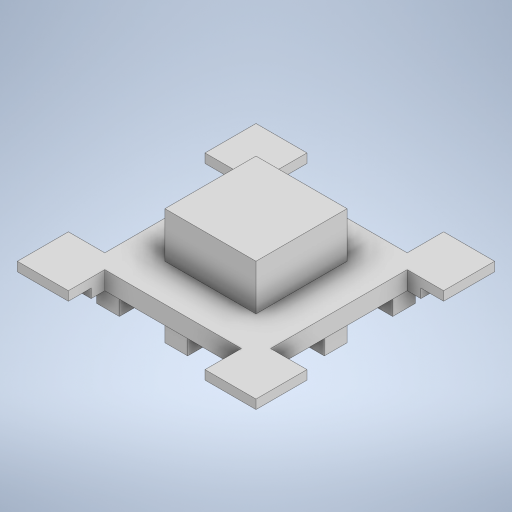
# Autodesk Inventor part: sensor_holder
Saved by Autodesk Inventor 2023.1 (Build 271208000, 208)
## iProperties
Created: 2022-08-08
Part Number: sensor_holder
Material: Generic
Document SubType Name: Modeling
Designer: fraaw
Density: 1 g/cm^3
Appearance: Default
Author: fraaw
## iProperties of the stored document sensor_holder_3DPrint.ipt
Created: 2022-08-08
Part Number: sensor_holder_3DPrint
Material: Generic
Document SubType Name: Modeling
Designer: fraaw
Density: 1 g/cm^3
Appearance: Default
Author: fraaw
Autodesk Inventor part; units mm, degrees
ref_plane "YZ Plane" through (0, 0, 0) normal (1, 0, 0) x (0, 1, 0)
ref_plane "XZ Plane" through (0, 0, 0) normal (0, 1, 0) x (-1, 0, 0)
ref_plane "XY Plane" through (0, 0, 0) normal (0, 0, 1) x (1, 0, 0)
sketch "Sketch1" plane through (0, 0, 0) normal (0, 1, 0) x (-1, 0, 0)
  line L0 (13.1, 13.1) -> (-13.1, 13.1)
  line L1 (-13.1, 13.1) -> (-13.1, -13.1)
  line L2 (-13.1, -13.1) -> (13.1, -13.1)
  line L3 (13.1, -13.1) -> (13.1, 13.1)
  line L4 (13.1, 13.1) -> (-13.1, -13.1) construction
  line L5 (-13.1, 13.1) -> (13.1, -13.1) construction
  point P0 (0, 0)
  dimension "d0" = 26.2
  dimension "d1" = 26.2
  constraints: 12 end point, 2 midpoint, 2 parallel, 1 horizontal, 1 perpendicular
  measures "d0" distance of L1.end L2.end
  measures "d1" distance of L2.end L0.start
extrude "Extrusion1" add sketch "Sketch1" along normal blind 1
sketch "Sketch3" plane through (0, 0, 0) normal (0, -1, 0) x (1, 0, 0)
  line L0 (-10.75, -10.75) -> (10.75, -10.75) construction
  line L1 (10.75, -10.75) -> (10.75, 10.75) construction
  line L2 (10.75, 10.75) -> (-10.75, 10.75) construction
  line L3 (-10.75, 10.75) -> (-10.75, -10.75) construction
  line L4 (-10.75, -10.75) -> (10.75, 10.75) construction
  line L5 (10.75, -10.75) -> (-10.75, 10.75) construction
  line L6 (-10.75, 10.75) -> (-4.25, 10.75) construction
  line L7 (-4.25, 10.75) -> (-4.25, 4.25) construction
  line L8 (-4.25, 4.25) -> (-10.75, 4.25) construction
  line L9 (-10.75, 4.25) -> (-10.75, 10.75) construction
  line L10 (-6.25, 6.25) -> (-8.75, 6.25)
  line L11 (-8.75, 6.25) -> (-8.75, 8.75)
  line L12 (-8.75, 8.75) -> (-6.25, 8.75)
  line L13 (-6.25, 8.75) -> (-6.25, 6.25)
  line L14 (-6.25, 6.25) -> (-8.75, 8.75) construction
  line L15 (-8.75, 6.25) -> (-6.25, 8.75) construction
  line L16 (-1.25, 8.75) -> (1.25, 8.75)
  line L17 (-1.25, 6.25) -> (-1.25, 8.75)
  line L18 (1.25, 6.25) -> (-1.25, 6.25)
  line L19 (1.25, 8.75) -> (1.25, 6.25)
  line L20 (6.25, 8.75) -> (8.75, 8.75)
  line L21 (6.25, 6.25) -> (6.25, 8.75)
  line L22 (8.75, 6.25) -> (6.25, 6.25)
  line L23 (8.75, 8.75) -> (8.75, 6.25)
  line L24 (-8.75, 1.25) -> (-6.25, 1.25)
  line L25 (-8.75, -1.25) -> (-8.75, 1.25)
  line L26 (-6.25, -1.25) -> (-8.75, -1.25)
  line L27 (-6.25, 1.25) -> (-6.25, -1.25)
  line L28 (-1.25, 1.25) -> (1.25, 1.25)
  line L29 (-1.25, -1.25) -> (-1.25, 1.25)
  line L30 (1.25, -1.25) -> (-1.25, -1.25)
  line L31 (1.25, 1.25) -> (1.25, -1.25)
  line L32 (6.25, 1.25) -> (8.75, 1.25)
  line L33 (6.25, -1.25) -> (6.25, 1.25)
  line L34 (8.75, -1.25) -> (6.25, -1.25)
  line L35 (8.75, 1.25) -> (8.75, -1.25)
  line L36 (-8.75, -6.25) -> (-6.25, -6.25)
  line L37 (-8.75, -8.75) -> (-8.75, -6.25)
  line L38 (-6.25, -8.75) -> (-8.75, -8.75)
  line L39 (-6.25, -6.25) -> (-6.25, -8.75)
  line L40 (-1.25, -6.25) -> (1.25, -6.25)
  line L41 (-1.25, -8.75) -> (-1.25, -6.25)
  line L42 (1.25, -8.75) -> (-1.25, -8.75)
  line L43 (1.25, -6.25) -> (1.25, -8.75)
  line L44 (6.25, -6.25) -> (8.75, -6.25)
  line L45 (6.25, -8.75) -> (6.25, -6.25)
  line L46 (8.75, -8.75) -> (6.25, -8.75)
  line L47 (8.75, -6.25) -> (8.75, -8.75)
  point P0 (0, 0)
  point P1 (-7.5, 7.5)
  dimension "d8" = 21.5
  dimension "d9" = 6.5
  dimension "d10" = 6.5
  dimension "d11" = 2.5
  dimension "d12" = 3.25
  dimension "d15" = 7.5
  dimension "d18" = 7.5
  constraints: 96 end point, 6 parallel, 4 horizontal, 4 midpoint, 3 perpendicular, 3 point on line, 1 vertical, 64 other
  measures "d8" distance of L1.end L2.end
  measures "d9" distance of L7.end L8.end
  measures "d10" distance of L6.end L7.end
  measures "d11" distance of L11.end L12.end
  measures "d12" distance from line of point (-7.5, 7.5) L9
  measures "d15" distance of L11.end L16.start
  measures "d18" distance of L11.end L24.start
extrude "Extrusion3" add sketch "Sketch3" along normal blind 3
sketch "Sketch5" plane through (0, 1, 0) normal (0, 1, 0) x (1, 0, 0)
  line L0 (-5, -5) -> (5, -5)
  line L1 (5, -5) -> (5, 5)
  line L2 (5, 5) -> (-5, 5)
  line L3 (-5, 5) -> (-5, -5)
  line L4 (-5, -5) -> (5, 5) construction
  line L5 (5, -5) -> (-5, 5) construction
  point P0 (0, 0)
  dimension "d23" = 10
  dimension "d24" = 10
  constraints: 12 end point, 2 midpoint, 2 parallel, 1 horizontal, 1 perpendicular
  measures "d23" distance of L1.end L2.end
  measures "d24" distance of L2.end L0.start
extrude "Extrusion4" add sketch "Sketch5" along normal blind 5
sketch "Sketch6" plane through (0, 0, 0) normal (0, -1, 0) x (1, 0, 0)
  line L0 (-10.6, 10.6) -> (10.6, 10.6)
  line L1 (10.6, 10.6) -> (10.6, -10.6)
  line L2 (10.6, -10.6) -> (-10.6, -10.6)
  line L3 (-10.6, -10.6) -> (-10.6, 10.6)
  line L4 (-10.6, 10.6) -> (10.6, -10.6) construction
  line L5 (10.6, 10.6) -> (-10.6, -10.6) construction
  point P0 (0, 0)
  dimension "d27" = 21.2
  dimension "d28" = 21.2
  constraints: 12 end point, 2 midpoint, 2 parallel, 1 horizontal, 1 perpendicular
  measures "d27" distance of L0.end L1.end
  measures "d28" distance of L0.start L0.end
extrude "Extrusion5" add sketch "Sketch6" along normal blind 1
sketch "Sketch7" plane through (0, -1, 0) normal (0, -1, 0) x (1, 0, 0)
  line L0 (-13.1, 13.1) -> (13.1, 13.1) projected
  line L1 (-7.5, 9.1) -> (7.5, 9.1)
  line L2 (7.5, 9.1) -> (7.5, 13.1)
  line L3 (7.5, 13.1) -> (-7.5, 13.1)
  line L4 (-7.5, 13.1) -> (-7.5, 9.1)
  line L5 (-7.5, 9.1) -> (7.5, 13.1) construction
  line L6 (7.5, 9.1) -> (-7.5, 13.1) construction
  line L7 (-9.1, 7.5) -> (-13.1, 7.5)
  line L8 (-13.1, 7.5) -> (-13.1, -7.5)
  line L9 (-9.1, -7.5) -> (-9.1, 7.5)
  line L10 (-13.1, -7.5) -> (-9.1, -7.5)
  line L11 (-7.5, -9.1) -> (-7.5, -13.1)
  line L12 (-7.5, -13.1) -> (7.5, -13.1)
  line L13 (7.5, -9.1) -> (-7.5, -9.1)
  line L14 (7.5, -13.1) -> (7.5, -9.1)
  line L15 (9.1, -7.5) -> (13.1, -7.5)
  line L16 (13.1, -7.5) -> (13.1, 7.5)
  line L17 (9.1, 7.5) -> (9.1, -7.5)
  line L18 (13.1, 7.5) -> (9.1, 7.5)
  point P0 (0, 0)
  point P1 (0, 11.1)
  dimension "d31" = 4
  dimension "d32" = 15
  dimension "d37" = 360
  constraints: 36 end point, 2 midpoint, 2 parallel, 1 horizontal, 1 perpendicular, 1 point on line, 33 other
  measures "d31" distance of L1.end L2.end
  measures "d32" distance of L1.start L1.end
extrude "Extrusion6" cut sketch "Sketch7" against normal up to surface (2 mm away)
equation "\"d1\" = d0"
equation "\"d10\" = d9"
equation "\"d12\" = 0.5 * d9"
equation "\"d24\" = d23"
equation "\"d28\" = d27"
body "Solid1"
